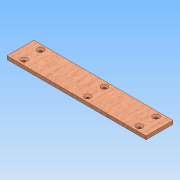
# Autodesk Inventor part: Top_Slider Piece 2
Saved by Autodesk Inventor 2018.1 (Build 221171000, 171)
## iProperties
Created: 2019-03-18
Part Number: Top_Slider Piece 2
Material: Wood (Oak)
Document SubType Name: Modeling
Designer: James
Density: 0.76 g/cm^3
Appearance: White Oak - Natural Medium Gloss
Author: James
Autodesk Inventor part; units mm, degrees
ref_plane "YZ Plane" through (0, 0, 0) normal (1, 0, 0) x (0, 1, 0)
ref_plane "XZ Plane" through (0, 0, 0) normal (0, 1, 0) x (-1, 0, 0)
ref_plane "XY Plane" through (0, 0, 0) normal (0, 0, 1) x (1, 0, 0)
sketch "Sketch1" plane through (0, 0, 0) normal (0, 0, 1) x (1, 0, 0)
  line L0 (0, 0) -> (207, 0)
  line L1 (207, 0) -> (207, 40)
  line L2 (207, 40) -> (0, 40)
  line L3 (0, 40) -> (0, 0)
  dimension "d0" = 207
  dimension "d1" = 40
  constraints: 8 end point, 2 parallel, 1 horizontal, 1 perpendicular
  measures "d0" distance of L2.end L1.end
  measures "d1" distance of L1.end L0.end
extrude "Extrusion1" add sketch "Sketch1" along normal blind 5
sketch "Sketch2" plane through (0, 0, 5) normal (0, 0, 1) x (1, 0, 0)
  line L0 (207, 40) -> (0, 40) projected
  line L1 (0, 0) -> (207, 0) projected
  line L2 (0, 40) -> (0, 0) projected
  point P0 (17.5, 32.5)
  point P1 (17.5, 7.5)
  point P2 (112.5, 32.5)
  point P3 (112.5, 7.5)
  point P4 (189.5, 32.5)
  point P5 (189.5, 7.5)
  dimension "d4" = 7.5
  dimension "d5" = 7.5
  dimension "d6" = 17.5
  dimension "d7" = 95
  dimension "d8" = 77
  constraints: 4 horizontal alignment, 3 vertical alignment
  measures "d4" distance from line of L0 point (17.5, 32.5)
  measures "d5" distance from line of L1 point (17.5, 7.5)
  measures "d6" distance from line of L2 point (17.5, 32.5)
  measures "d7" distance of point (17.5, 32.5) point (112.5, 32.5)
  measures "d8" distance of point (189.5, 32.5) point (112.5, 32.5)
hole "Hole1" at (17.5, 32.5, 5) at (17.5, 7.5, 5) at (112.5, 32.5, 5) at (112.5, 7.5, 5) at (189.5, 32.5, 5) at (189.5, 7.5, 5) direction (0, 0, -1) diameter 4.5 end through all countersink diameter 9.4 countersink angle 90 clearance for "Flat Head Machine Screw" size "M4" standard "Ansi Metric M Profile"
equation "\"d5\" = d4"
body "Solid1"
